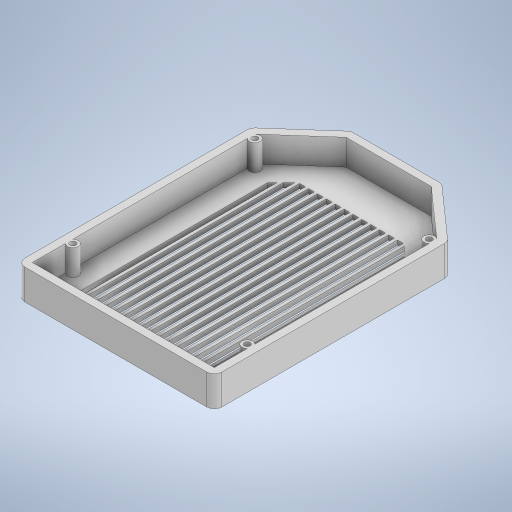
# Autodesk Inventor part: Pieza5
Saved by Autodesk Inventor 2024.3 (Build 283343000, 343)
## iProperties
Created: 2025-02-01
Part Number: Pieza5
Material: Genérico
Document SubType Name: Modeling
Designer: Jorge
Density: 1 g/cm^3
Appearance: Valor por defecto
Author: Jorge
Autodesk Inventor part; units mm, degrees
ref_plane "YZ Plane" through (0, 0, 0) normal (1, 0, 0) x (0, 1, 0)
ref_plane "XY Plane" through (0, 0, 0) normal (0, 0, 1) x (1, 0, 0)
sketch "Boceto1" plane through (0, 0, 0) normal (0, 1, 0) x (-1, 0, 0)
  line L0 (0, 0) -> (0, -154)
  line L1 (35, -185) -> (95, -185)
  line L2 (130, -154) -> (130, 0)
  line L3 (130, 0) -> (0, 0)
  line L4 (0, 0) -> (0, -154) construction
  line L5 (65, -185) -> (95, -185) construction
  line L6 (95, -185) -> (95, -206.4869) construction
  line L7 (95, -206.4869) -> (35, -206.4869) construction
  line L8 (35, -206.4869) -> (35, -185) construction
  line L9 (0, -154) -> (35, -185)
  line L10 (95, -185) -> (130, -154)
  line L11 (61.4516, 0) -> (61.4516, -5) construction
  line L12 (130, -81.3037) -> (125, -81.3037) construction
  line L13 (0, -85.0807) -> (5, -85.0807) construction
  line L14 (125, -5) -> (5, -5)
  line L15 (5, -5) -> (5, -148.3548)
  line L16 (125, -148.3548) -> (125, -5)
  line L17 (112.5, -169.5) -> (109.1848, -165.7571) construction
  line L18 (65, -185) -> (65, -180) construction
  line L19 (17.5, -169.5) -> (20.8152, -165.7571) construction
  line L20 (20.8152, -165.7571) -> (5, -151.7493)
  line L21 (20.8152, -165.7571) -> (36.8959, -180)
  line L22 (36.8959, -180) -> (93.1041, -180)
  line L23 (93.1041, -180) -> (125, -151.7493)
  line L24 (125, -151.7493) -> (125, -148.3548)
  line L25 (5, -148.3548) -> (5, -151.7493)
  dimension "d2" = 154
  dimension "d3" = 30
  dimension "d4" = 60
  dimension "d5" = 5
  dimension "d6" = 5
  dimension "d7" = 5
  dimension "d8" = 5
  dimension "d9" = 5
  dimension "d10" = 5
  constraints: 52 end point, 9 perpendicular, 4 horizontal, 3 midpoint, 3 point on line, 3 vertical, 2 parallel
  measures "d2" distance of L0.end L0.start
  measures "d3" distance of L1.end L5.start
  measures "d4" distance of L6.end L7.end
  measures "d5" distance of L11.start L11.end
  measures "d6" distance of L12.start L12.end
  measures "d7" distance of L13.start L13.end
  measures "d8" distance of L17.start L17.end
  measures "d9" distance of L5.start L18.end
  measures "d10" distance of L19.start L19.end
extrude "Extrusión1" add sketch "Boceto1" along normal blind 3 contours L16 L24 L23 L22 L21 L20 L25 L15 L14
extrude "Extrusión2" add sketch "Boceto1" along normal blind 20
ref_plane "Plano de trabajo1" through (0, 20, 0) normal (0, 1, 0) x (-1, 0, 0)
sketch "Boceto2" plane through (0, 20, 0) normal (0, 1, 0) x (-1, 0, 0)
  line L0 (0, 0) -> (0, -154) construction
  line L1 (0, 0) -> (0, -26.749) construction
  line L2 (130, -154) -> (130, 0) construction
  line L3 (125, -151.7493) -> (93.1041, -180) construction
  line L4 (125, -151.7493) -> (5, -151.7493) construction
  line L5 (65, -151.7493) -> (65, -26.749) construction
  line L6 (125, -89.2492) -> (5, -89.2492) construction
  line L7 (5, -151.7493) -> (5, -5) construction
  line L8 (125, -26.749) -> (125, -31.749) construction
  line L9 (125, -31.749) -> (120, -31.749) construction
  line L10 (120, -31.749) -> (120, -26.749) construction
  line L11 (125, -31.749) -> (120, -26.749) construction
  line L12 (120, -31.749) -> (125, -26.749) construction
  circle A0 centre (122.5, -29.249) radius 2
  line L13 (125, -31.749) -> (125, -26.749)
  arc A1 (120, -26.749) -> (125, -31.749) centre (122.5, -29.249) ccw
  line L14 (5, -26.749) -> (5, -31.749) construction
  circle A2 centre (7.5, -29.249) radius 2
  line L15 (5, -31.749) -> (5, -26.749)
  arc A3 (5, -31.749) -> (10, -26.749) centre (7.5, -29.249) ccw
  arc A4 (125, -26.749) -> (120.5, -32.1645) centre (122.5, -29.249) ccw
  arc A5 (10.6306, -27.606) -> (5, -26.749) centre (7.5, -29.249) ccw
  line L16 (5, -26.749) -> (5, -173.4983) construction
  line L17 (125, -151.7493) -> (125, -146.7493) construction
  line L18 (120, -146.7493) -> (125, -151.7493) construction
  circle A6 centre (122.5, -149.2493) radius 2
  line L19 (125, -146.7493) -> (125, -151.7493)
  arc A7 (125, -146.7493) -> (120, -151.7493) centre (122.5, -149.2493) ccw
  arc A8 (10, -151.7493) -> (5, -146.7493) centre (7.5, -149.2493) ccw
  line L20 (5, -151.7493) -> (5, -146.7493) construction
  line L21 (5, -146.7493) -> (5, -151.7493)
  circle A9 centre (7.5, -149.2493) radius 2
  arc A10 (120.5, -146.3339) -> (125, -151.7493) centre (122.5, -149.2493) ccw
  arc A11 (5, -151.7493) -> (10.6306, -150.8923) centre (7.5, -149.2493) ccw
  point P0 (10, -151.7493)
  point P1 (10, -26.749)
  point P2 (120, -26.749)
  dimension "d16" = 26.749
  dimension "d19" = 4
  constraints: 36 end point, 21 symmetric about line, 20 point on circle, 12 centre point, 8 coincident, 2 midpoint, 2 perpendicular, 2 point on line, 1 horizontal, 8 other
  measures "d16" distance of L0.start L1.end
  measures "d19" diameter of A0
extrude "Extrusión3" add sketch "Boceto2" against normal blind 17
extrude "Extrusión4" cut sketch "Boceto2" against normal through all contours A0 | A2 | A6 | A9
sketch "Boceto3" plane through (0, 3, 0) normal (0, 1, 0) x (1, 0, 0)
  line L0 (-125, 5) -> (-5, 5) construction
  line L1 (-65, 5) -> (-110, 5) construction
  line L2 (-110, 5) -> (-110, 15) construction
  line L3 (-110, 15) -> (-20, 15)
  line L4 (-20, 15) -> (-20, 145.2684)
  line L5 (-30, 155.2684) -> (-100, 155.2684)
  line L6 (-110, 145.2684) -> (-110, 15)
  line L7 (-65, 15) -> (-65, 155.2684) construction
  line L8 (-100, 155.2684) -> (-110, 145.2684)
  line L9 (-30, 155.2684) -> (-20, 145.2684)
  line L10 (-106.9205, 15) -> (-104.9205, 15)
  line L11 (-104.9205, 15) -> (-104.9205, 155.2684)
  line L12 (-106.9205, 155.2684) -> (-106.9205, 15)
  line L13 (-99.0505, 15) -> (-99.0505, 155.2684)
  line L14 (-101.0505, 155.2684) -> (-101.0505, 15)
  line L15 (-93.1805, 15) -> (-93.1805, 155.2684)
  line L16 (-95.1805, 155.2684) -> (-95.1805, 15)
  line L17 (-87.3105, 15) -> (-87.3105, 155.2684)
  line L18 (-89.3105, 155.2684) -> (-89.3105, 15)
  line L19 (-81.4405, 15) -> (-81.4405, 155.2684)
  line L20 (-83.4405, 155.2684) -> (-83.4405, 15)
  line L21 (-75.5705, 15) -> (-75.5705, 155.2684)
  line L22 (-77.5705, 155.2684) -> (-77.5705, 15)
  line L23 (-69.7005, 15) -> (-69.7005, 155.2684)
  line L24 (-71.7005, 155.2684) -> (-71.7005, 15)
  line L25 (-63.8305, 15) -> (-63.8305, 155.2684)
  line L26 (-65.8305, 155.2684) -> (-65.8305, 15)
  line L27 (-57.9605, 15) -> (-57.9605, 155.2684)
  line L28 (-59.9605, 155.2684) -> (-59.9605, 15)
  line L29 (-52.0905, 15) -> (-52.0905, 155.2684)
  line L30 (-54.0905, 155.2684) -> (-54.0905, 15)
  line L31 (-46.2205, 15) -> (-46.2205, 155.2684)
  line L32 (-48.2205, 155.2684) -> (-48.2205, 15)
  line L33 (-40.3505, 15) -> (-40.3505, 155.2684)
  line L34 (-42.3505, 155.2684) -> (-42.3505, 15)
  line L35 (-34.4805, 15) -> (-34.4805, 155.2684)
  line L36 (-36.4805, 155.2684) -> (-36.4805, 15)
  line L37 (-28.6105, 15) -> (-28.6105, 155.2684)
  line L38 (-30.6105, 155.2684) -> (-30.6105, 15)
  line L39 (-22.7405, 15) -> (-22.7405, 155.2684)
  line L40 (-24.7405, 155.2684) -> (-24.7405, 15)
  line L41 (-106.9205, 148.348) -> (-104.9205, 150.348)
  line L42 (-101.0505, 154.218) -> (-100, 155.2684)
  line L43 (-110, 145.2684) -> (-100, 155.2684)
  line L44 (-100, 155.2684) -> (-30, 155.2684)
  line L45 (-30, 155.2684) -> (-20, 145.2684)
  line L46 (-20, 145.2684) -> (-20, 15)
  line L47 (-110, 15) -> (-20, 15)
  line L48 (-110, 15) -> (-110, 145.2684)
  line L49 (-83.4405, 15) -> (-81.4405, 15)
  line L50 (-77.5705, 15) -> (-75.5705, 15)
  line L51 (-87.3105, 15) -> (-89.3105, 15)
  line L52 (-93.1805, 15) -> (-95.1805, 15)
  line L53 (-99.0505, 15) -> (-101.0505, 15)
  line L54 (-104.9205, 15) -> (-106.9205, 15)
  line L55 (-71.7005, 15) -> (-69.7005, 15)
  line L56 (-65.8305, 15) -> (-63.8305, 15)
  line L57 (-59.9605, 15) -> (-57.9605, 15)
  line L58 (-54.0905, 15) -> (-52.0905, 15)
  line L59 (-48.2205, 15) -> (-46.2205, 15)
  line L60 (-42.3505, 15) -> (-40.3505, 15)
  line L61 (-36.4805, 15) -> (-34.4805, 15)
  line L62 (-30.6105, 15) -> (-28.6105, 15)
  line L63 (-24.7405, 15) -> (-22.7405, 15)
  line L64 (-22.7405, 148.0089) -> (-24.7405, 150.0089)
  line L65 (-28.6105, 153.8789) -> (-30, 155.2684)
  line L66 (-30.6105, 155.2684) -> (-30, 155.2684)
  line L67 (-35, 185) -> (-95, 185) projected
  line L68 (-34.4805, 155.2684) -> (-36.4805, 155.2684)
  line L69 (-40.3505, 155.2684) -> (-42.3505, 155.2684)
  line L70 (-46.2205, 155.2684) -> (-48.2205, 155.2684)
  line L71 (-52.0905, 155.2684) -> (-54.0905, 155.2684)
  line L72 (-57.9605, 155.2684) -> (-59.9605, 155.2684)
  line L73 (-63.8305, 155.2684) -> (-65.8305, 155.2684)
  line L74 (-69.7005, 155.2684) -> (-71.7005, 155.2684)
  line L75 (-75.5705, 155.2684) -> (-77.5705, 155.2684)
  line L76 (-81.4405, 155.2684) -> (-83.4405, 155.2684)
  line L77 (-87.3105, 155.2684) -> (-89.3105, 155.2684)
  line L78 (-93.1805, 155.2684) -> (-95.1805, 155.2684)
  line L79 (-99.0505, 155.2684) -> (-100, 155.2684)
  line L80 (-101.0505, 154.218) -> (-100, 155.2684)
  line L81 (-104.9205, 150.348) -> (-106.9205, 148.348)
  line L82 (-106.9205, 148.348) -> (-104.9205, 150.348)
  point P0 (0, 0)
  dimension "d24" = 45
  dimension "d25" = 10
  dimension "d32" = 5.87
  constraints: 158 end point, 56 horizontal alignment, 33 parallel, 23 collinear, 13 point on line, 10 horizontal, 4 perpendicular, 2 symmetric about line, 2 vertical, 1 midpoint, 9 other
  measures "d24" distance of L1.start L1.end
  measures "d25" distance of L1.end L2.end
  measures "d32" distance of L10.end L13.start
extrude "Extrusión5" cut sketch "Boceto3" against normal blind 10 contours L6 L8 L12 L3 | L11 L8 L14 L3 | L13 L5 L16 L3 | L15 L5 L18 L3 | L17 L5 L20 L3 | L19 L5 L22 L3 | L21 L5 L24 L3 | L23 L5 L26 L3 | L25 L5 L28 L3 | L27 L5 L30 L3 | L29 L5 L32 L3 | L31 L5 L34 L3 | L33 L5 L36 L3 | L35 L5 L38 L3 | L37 L9 L40 L3 | L39 L9 L4 L3
fillet "Empalme1" radius 5 4 edges at (-130, 10, 0) (0, 10, 0) (0, 10, -154) (-130, 10, -154)
fillet "Empalme2" radius 5 2 edges at (-95, 10, -185) (-35, 10, -185)
